Autodesk Inventor part; units mm, degrees
(part 4 of 6)
  line L818 (127.9253, -63.5518) -> (127.9253, -44.4306)
  spline S858 degree 2 poles (127.9253, -44.4306) (127.9253, -44.0268) (128.4872, -43.4824) (128.8735, -43.4824) knots 0 0 0 1 2 2 2
  spline S859 degree 2 poles (128.8735, -43.4824) (129.2773, -43.4824) (129.5583, -43.7458) knots 0 0 0 1 1 1
  spline S860 degree 2 poles (129.5583, -43.7458) (129.6636, -43.8512) (129.7163, -43.9741) knots 0 0 0 1 1 1
  line L819 (129.7163, -43.9741) -> (136.845, -59.2676)
  line L820 (136.845, -59.2676) -> (136.845, -44.4306)
  spline S861 degree 2 poles (136.845, -44.4306) (136.845, -44.0268) (137.3894, -43.4824) (137.7932, -43.4824) knots 0 0 0 1 2 2 2
  spline S862 degree 2 poles (137.7932, -43.4824) (138.197, -43.4824) (138.7414, -44.0268) (138.7414, -44.4306) knots 0 0 0 1 2 2 2
  line L821 (138.7414, -44.4306) -> (138.7414, -63.5694)
  spline S863 degree 2 poles (138.7414, -63.5694) (138.7414, -63.9381) (138.478, -64.2191) knots 0 0 0 1 1 1
  spline S864 degree 2 poles (138.478, -64.2191) (138.197, -64.5) (137.7932, -64.5) knots 0 0 0 1 1 1
  spline S865 degree 2 poles (137.7932, -64.5) (137.3894, -64.5) (137.126, -64.2191) knots 0 0 0 1 1 1
  spline S866 degree 2 poles (137.126, -64.2191) (136.9855, -64.0786) (136.8802, -63.8679) knots 0 0 0 1 1 1
  line L822 (136.8802, -63.8679) -> (129.8392, -48.6271)
  line L823 (129.8392, -48.6271) -> (129.8392, -63.5518)
  spline S867 degree 2 poles (165.7097, -44.4482) (165.7097, -44.0443) (166.2716, -43.5) (166.6579, -43.5) knots 0 0 0 1 2 2 2
  spline S868 degree 2 poles (166.6579, -43.5) (167.0617, -43.5) (167.6236, -44.0443) (167.6236, -44.4482) knots 0 0 0 1 2 2 2
  line L824 (167.6236, -44.4482) -> (167.6236, -63.5518)
  spline S869 degree 2 poles (167.6236, -63.5518) (167.6236, -63.9381) (167.0617, -64.5) (166.6579, -64.5) knots 0 0 0 1 2 2 2
  spline S870 degree 2 poles (166.6579, -64.5) (166.2716, -64.5) (165.7097, -63.9381) (165.7097, -63.5518) knots 0 0 0 1 2 2 2
  line L825 (165.7097, -63.5518) -> (165.7097, -44.4482)
  spline S871 degree 2 poles (-166.6579, -94.1789) (-166.2716, -94.1789) (-165.7097, -94.7408) (-165.7097, -95.1446) knots 0 0 0 1 2 2 2
  spline S872 degree 2 poles (-165.7097, -95.1446) (-165.7097, -95.5309) (-166.2716, -96.0928) (-166.6579, -96.0928) knots 0 0 0 1 2 2 2
  line L826 (-166.6579, -96.0928) -> (-169.836, -96.0928)
  line L827 (-169.836, -96.0928) -> (-170.8017, -99.7099)
  spline S873 degree 2 poles (-170.8017, -99.7099) (-170.8895, -100.0084) (-171.0826, -100.2191) knots 0 0 0 1 1 1
  spline S874 degree 2 poles (-171.0826, -100.2191) (-171.3636, -100.5) (-171.7499, -100.5) knots 0 0 0 1 1 1
  spline S875 degree 2 poles (-171.7499, -100.5) (-172.1537, -100.5) (-172.7156, -99.9381) (-172.7156, -99.5518) knots 0 0 0 1 2 2 2
  spline S876 degree 2 poles (-172.7156, -99.5518) (-172.7156, -99.4289) (-172.698, -99.3411) knots 0 0 0 1 1 1
  line L828 (-172.698, -99.3411) -> (-167.606, -80.3428)
  spline S877 degree 2 poles (-167.606, -80.3428) (-167.5358, -80.0268) (-167.3251, -79.7985) knots 0 0 0 1 1 1
  spline S878 degree 2 poles (-167.3251, -79.7985) (-167.0442, -79.5) (-166.6579, -79.5) knots 0 0 0 1 1 1
  spline S879 degree 2 poles (-166.6579, -79.5) (-166.2716, -79.5) (-165.9731, -79.7985) knots 0 0 0 1 1 1
  spline S880 degree 2 poles (-165.9731, -79.7985) (-165.7975, -80.0268) (-165.7273, -80.3428) knots 0 0 0 1 1 1
  line L829 (-165.7273, -80.3428) -> (-160.6353, -99.3411)
  spline S881 degree 2 poles (-160.6353, -99.3411) (-160.6178, -99.4289) (-160.6178, -99.5518) knots 0 0 0 1 1 1
  spline S882 degree 2 poles (-160.6178, -99.5518) (-160.6178, -99.9381) (-161.1796, -100.5) (-161.5659, -100.5) knots 0 0 0 1 2 2 2
  spline S883 degree 2 poles (-161.5659, -100.5) (-161.9698, -100.5) (-162.2331, -100.2191) knots 0 0 0 1 1 1
  spline S884 degree 2 poles (-162.2331, -100.2191) (-162.4438, -100.0084) (-162.5316, -99.7099) knots 0 0 0 1 1 1
  line L830 (-162.5316, -99.7099) -> (-166.6579, -84.2057)
  line L831 (-166.6579, -84.2057) -> (-169.3268, -94.1789)
  line L832 (-169.3268, -94.1789) -> (-166.6579, -94.1789)
  spline S885 degree 2 poles (-130.524, -97.7784) (-130.2606, -97.5151) (-129.8567, -97.5151) knots 0 0 0 1 1 1
  spline S886 degree 2 poles (-129.8567, -97.5151) (-129.4705, -97.5151) (-128.9086, -98.0594) (-128.9086, -98.4632) knots 0 0 0 1 2 2 2
  spline S887 degree 2 poles (-128.9086, -98.4632) (-128.9086, -98.8495) (-129.172, -99.1304) knots 0 0 0 1 1 1
  spline S888 degree 2 poles (-129.172, -99.1304) (-130.524, -100.5) (-132.3676, -100.5) knots 0 0 0 1 1 1
  spline S889 degree 2 poles (-132.3676, -100.5) (-134.2288, -100.5) (-136.8275, -97.8838) (-136.8275, -96.0401) knots 0 0 0 1 2 2 2
  line L833 (-136.8275, -96.0401) -> (-136.8275, -83.2751)
  spline S890 degree 2 poles (-136.8275, -83.2751) (-136.8275, -81.4314) (-134.2288, -78.8152) (-132.3676, -78.8152) knots 0 0 0 1 2 2 2
  spline S891 degree 2 poles (-132.3676, -78.8152) (-130.524, -78.8152) (-129.172, -80.1848) knots 0 0 0 1 1 1
  spline S892 degree 2 poles (-129.172, -80.1848) (-128.9086, -80.4833) (-128.9086, -80.852) knots 0 0 0 1 1 1
  spline S893 degree 2 poles (-128.9086, -80.852) (-128.9086, -81.2559) (-129.4705, -81.8177) (-129.8567, -81.8177) knots 0 0 0 1 2 2 2
  spline S894 degree 2 poles (-129.8567, -81.8177) (-130.2606, -81.8177) (-130.524, -81.5368) knots 0 0 0 1 1 1
  spline S895 degree 2 poles (-130.524, -81.5368) (-131.3317, -80.7467) (-132.3676, -80.7467) knots 0 0 0 1 1 1
  spline S896 degree 2 poles (-132.3676, -80.7467) (-133.4387, -80.7467) (-134.9136, -82.2391) (-134.9136, -83.2926) knots 0 0 0 1 2 2 2
  line L834 (-134.9136, -83.2926) -> (-134.9136, -96.0226)
  spline S897 degree 2 poles (-134.9136, -96.0226) (-134.9136, -97.0761) (-133.4387, -98.5686) (-132.3676, -98.5686) knots 0 0 0 1 2 2 2
  spline S898 degree 2 poles (-132.3676, -98.5686) (-131.3317, -98.5686) (-130.524, -97.7784) knots 0 0 0 1 1 1
  spline S899 degree 2 poles (-104.7759, -80.4482) (-104.7759, -80.0443) (-104.214, -79.5) (-103.8278, -79.5) knots 0 0 0 1 2 2 2
  spline S900 degree 2 poles (-103.8278, -79.5) (-103.4239, -79.5) (-102.862, -80.0443) (-102.862, -80.4482) knots 0 0 0 1 2 2 2
  line L835 (-102.862, -80.4482) -> (-102.862, -89.0343)
  line L836 (-102.862, -89.0343) -> (-97.1555, -89.0343)
  line L837 (-97.1555, -89.0343) -> (-97.1555, -80.4482)
  spline S901 degree 2 poles (-97.1555, -80.4482) (-97.1555, -80.0443) (-96.5936, -79.5) (-96.1898, -79.5) knots 0 0 0 1 2 2 2
  spline S902 degree 2 poles (-96.1898, -79.5) (-95.8035, -79.5) (-95.2416, -80.0443) (-95.2416, -80.4482) knots 0 0 0 1 2 2 2
  line L838 (-95.2416, -80.4482) -> (-95.2416, -99.5518)
  spline S903 degree 2 poles (-95.2416, -99.5518) (-95.2416, -99.9381) (-95.8035, -100.5) (-96.1898, -100.5) knots 0 0 0 1 2 2 2
  spline S904 degree 2 poles (-96.1898, -100.5) (-96.5936, -100.5) (-97.1555, -99.9381) (-97.1555, -99.5518) knots 0 0 0 1 2 2 2
  line L839 (-97.1555, -99.5518) -> (-97.1555, -90.9482)
  line L840 (-97.1555, -90.9482) -> (-102.862, -90.9482)
  line L841 (-102.862, -90.9482) -> (-102.862, -99.5518)
  spline S905 degree 2 poles (-102.862, -99.5518) (-102.862, -99.9381) (-103.4239, -100.5) (-103.8278, -100.5) knots 0 0 0 1 2 2 2
  spline S906 degree 2 poles (-103.8278, -100.5) (-104.214, -100.5) (-104.7759, -99.9381) (-104.7759, -99.5518) knots 0 0 0 1 2 2 2
  line L842 (-104.7759, -99.5518) -> (-104.7759, -80.4482)
  spline S907 degree 2 poles (-70.3364, -81.3963) (-70.7227, -81.3963) (-71.2846, -80.852) (-71.2846, -80.4482) knots 0 0 0 1 2 2 2
  spline S908 degree 2 poles (-71.2846, -80.4482) (-71.2846, -80.0443) (-70.7227, -79.5) (-70.3364, -79.5) knots 0 0 0 1 2 2 2
  line L843 (-70.3364, -79.5) -> (-63.3305, -79.5)
  spline S909 degree 2 poles (-63.3305, -79.5) (-62.9267, -79.5) (-62.3648, -80.0443) (-62.3648, -80.4482) knots 0 0 0 1 2 2 2
  spline S910 degree 2 poles (-62.3648, -80.4482) (-62.3648, -80.852) (-62.9267, -81.3963) (-63.3305, -81.3963) knots 0 0 0 1 2 2 2
  line L844 (-63.3305, -81.3963) -> (-65.8765, -81.3963)
  line L845 (-65.8765, -81.3963) -> (-65.8765, -99.5518)
  spline S911 degree 2 poles (-65.8765, -99.5518) (-65.8765, -99.9381) (-66.4208, -100.5) (-66.8247, -100.5) knots 0 0 0 1 2 2 2
  spline S912 degree 2 poles (-66.8247, -100.5) (-67.2285, -100.5) (-67.7904, -99.9381) (-67.7904, -99.5518) knots 0 0 0 1 2 2 2
  line L846 (-67.7904, -99.5518) -> (-67.7904, -81.3963)
  line L847 (-67.7904, -81.3963) -> (-70.3364, -81.3963)
  spline S913 degree 2 poles (-34.2903, -80.4482) (-34.2903, -80.0443) (-33.7284, -79.5) (-33.3421, -79.5) knots 0 0 0 1 2 2 2
  spline S914 degree 2 poles (-33.3421, -79.5) (-32.9383, -79.5) (-32.3764, -80.0443) (-32.3764, -80.4482) knots 0 0 0 1 2 2 2
  line L848 (-32.3764, -80.4482) -> (-32.3764, -99.5518)
  spline S915 degree 2 poles (-32.3764, -99.5518) (-32.3764, -99.9381) (-32.9383, -100.5) (-33.3421, -100.5) knots 0 0 0 1 2 2 2
  spline S916 degree 2 poles (-33.3421, -100.5) (-33.7284, -100.5) (-34.2903, -99.9381) (-34.2903, -99.5518) knots 0 0 0 1 2 2 2
  line L849 (-34.2903, -99.5518) -> (-34.2903, -80.4482)
  spline S917 degree 2 poles (-3.4941, -99.5518) (-3.4941, -99.9381) (-4.056, -100.5) (-4.4599, -100.5) knots 0 0 0 1 2 2 2
  spline S918 degree 2 poles (-4.4599, -100.5) (-4.8462, -100.5) (-5.408, -99.9381) (-5.408, -99.5518) knots 0 0 0 1 2 2 2
  line L850 (-5.408, -99.5518) -> (-5.408, -80.4306)
  spline S919 degree 2 poles (-5.408, -80.4306) (-5.408, -80.0268) (-4.8462, -79.4824) (-4.4599, -79.4824) knots 0 0 0 1 2 2 2
  spline S920 degree 2 poles (-4.4599, -79.4824) (-4.056, -79.4824) (-3.7751, -79.7458) knots 0 0 0 1 1 1
  spline S921 degree 2 poles (-3.7751, -79.7458) (-3.6697, -79.8512) (-3.6171, -79.9741) knots 0 0 0 1 1 1
  line L851 (-3.6171, -79.9741) -> (3.5117, -95.2676)
  line L852 (3.5117, -95.2676) -> (3.5117, -80.4306)
  spline S922 degree 2 poles (3.5117, -80.4306) (3.5117, -80.0268) (4.056, -79.4824) (4.4599, -79.4824) knots 0 0 0 1 2 2 2
  spline S923 degree 2 poles (4.4599, -79.4824) (4.8637, -79.4824) (5.408, -80.0268) (5.408, -80.4306) knots 0 0 0 1 2 2 2
  line L853 (5.408, -80.4306) -> (5.408, -99.5694)
  spline S924 degree 2 poles (5.408, -99.5694) (5.408, -99.9381) (5.1446, -100.2191) knots 0 0 0 1 1 1
  spline S925 degree 2 poles (5.1446, -100.2191) (4.8637, -100.5) (4.4599, -100.5) knots 0 0 0 1 1 1
  spline S926 degree 2 poles (4.4599, -100.5) (4.056, -100.5) (3.7926, -100.2191) knots 0 0 0 1 1 1
  spline S927 degree 2 poles (3.7926, -100.2191) (3.6522, -100.0786) (3.5468, -99.8679) knots 0 0 0 1 1 1
  line L854 (3.5468, -99.8679) -> (-3.4941, -84.6271)
  line L855 (-3.4941, -84.6271) -> (-3.4941, -99.5518)
  spline S928 degree 2 poles (28.8822, -80.1497) (28.8822, -79.7458) (29.4441, -79.1839) (29.8304, -79.1839) knots 0 0 0 1 2 2 2
  spline S929 degree 2 poles (29.8304, -79.1839) (30.2343, -79.1839) (30.7961, -79.7458) (30.7961, -80.1497) knots 0 0 0 1 2 2 2
  line L856 (30.7961, -80.1497) -> (30.7961, -96.0401)
  spline S930 degree 2 poles (30.7961, -96.0401) (30.7961, -97.0936) (32.2886, -98.5861) (33.3421, -98.5861) knots 0 0 0 1 2 2 2
  spline S931 degree 2 poles (33.3421, -98.5861) (34.3956, -98.5861) (35.8881, -97.0936) (35.8881, -96.0401) knots 0 0 0 1 2 2 2
  line L857 (35.8881, -96.0401) -> (35.8881, -80.1497)
  spline S932 degree 2 poles (35.8881, -80.1497) (35.8881, -79.7458) (36.4324, -79.1839) (36.8363, -79.1839) knots 0 0 0 1 2 2 2
  spline S933 degree 2 poles (36.8363, -79.1839) (37.2401, -79.1839) (37.802, -79.7458) (37.802, -80.1497) knots 0 0 0 1 2 2 2
  line L858 (37.802, -80.1497) -> (37.802, -96.0401)
  spline S934 degree 2 poles (37.802, -96.0401) (37.802, -97.8838) (35.1858, -100.5) (33.3421, -100.5) knots 0 0 0 1 2 2 2
  spline S935 degree 2 poles (33.3421, -100.5) (31.4985, -100.5) (28.8822, -97.8838) (28.8822, -96.0401) knots 0 0 0 1 2 2 2
  line L859 (28.8822, -96.0401) -> (28.8822, -80.1497)
  spline S936 degree 2 poles (31.0244, -74.0744) (31.5511, -74.0744) (32.3062, -74.8294) (32.3062, -75.3562) knots 0 0 0 1 2 2 2
  spline S937 degree 2 poles (32.3062, -75.3562) (32.3062, -75.8829) (31.5511, -76.6204) (31.0244, -76.6204) knots 0 0 0 1 2 2 2
  spline S938 degree 2 poles (31.0244, -76.6204) (30.4976, -76.6204) (29.7602, -75.8829) (29.7602, -75.3562) knots 0 0 0 1 2 2 2
  spline S939 degree 2 poles (29.7602, -75.3562) (29.7602, -74.8294) (30.4976, -74.0744) (31.0244, -74.0744) knots 0 0 0 1 2 2 2
  spline S940 degree 2 poles (35.6598, -74.0744) (36.1866, -74.0744) (36.9416, -74.8294) (36.9416, -75.3562) knots 0 0 0 1 2 2 2
  spline S941 degree 2 poles (36.9416, -75.3562) (36.9416, -75.8829) (36.1866, -76.6204) (35.6598, -76.6204) knots 0 0 0 1 2 2 2
  spline S942 degree 2 poles (35.6598, -76.6204) (35.1331, -76.6204) (34.3956, -75.8829) (34.3956, -75.3562) knots 0 0 0 1 2 2 2
  spline S943 degree 2 poles (34.3956, -75.3562) (34.3956, -74.8294) (35.1331, -74.0744) (35.6598, -74.0744) knots 0 0 0 1 2 2 2
  spline S944 degree 2 poles (63.1725, -99.5518) (63.1725, -99.9381) (62.6106, -100.5) (62.2068, -100.5) knots 0 0 0 1 2 2 2
  spline S945 degree 2 poles (62.2068, -100.5) (61.8205, -100.5) (61.2586, -99.9381) (61.2586, -99.5518) knots 0 0 0 1 2 2 2
  line L860 (61.2586, -99.5518) -> (61.2586, -80.4306)
  spline S946 degree 2 poles (61.2586, -80.4306) (61.2586, -80.0268) (61.8205, -79.4824) (62.2068, -79.4824) knots 0 0 0 1 2 2 2
  spline S947 degree 2 poles (62.2068, -79.4824) (62.6106, -79.4824) (62.8916, -79.7458) knots 0 0 0 1 1 1
  spline S948 degree 2 poles (62.8916, -79.7458) (62.9969, -79.8512) (63.0496, -79.9741) knots 0 0 0 1 1 1
  line L861 (63.0496, -79.9741) -> (70.1784, -95.2676)
  line L862 (70.1784, -95.2676) -> (70.1784, -80.4306)
  spline S949 degree 2 poles (70.1784, -80.4306) (70.1784, -80.0268) (70.7227, -79.4824) (71.1265, -79.4824) knots 0 0 0 1 2 2 2
  spline S950 degree 2 poles (71.1265, -79.4824) (71.5304, -79.4824) (72.0747, -80.0268) (72.0747, -80.4306) knots 0 0 0 1 2 2 2
  line L863 (72.0747, -80.4306) -> (72.0747, -99.5694)
  spline S951 degree 2 poles (72.0747, -99.5694) (72.0747, -99.9381) (71.8113, -100.2191) knots 0 0 0 1 1 1
  spline S952 degree 2 poles (71.8113, -100.2191) (71.5304, -100.5) (71.1265, -100.5) knots 0 0 0 1 1 1
  spline S953 degree 2 poles (71.1265, -100.5) (70.7227, -100.5) (70.4593, -100.2191) knots 0 0 0 1 1 1
  spline S954 degree 2 poles (70.4593, -100.2191) (70.3188, -100.0786) (70.2135, -99.8679) knots 0 0 0 1 1 1
  line L864 (70.2135, -99.8679) -> (63.1725, -84.6271)
  line L865 (63.1725, -84.6271) -> (63.1725, -99.5518)
  spline S955 degree 2 poles (99.0431, -80.4482) (99.0431, -80.0443) (99.6049, -79.5) (99.9912, -79.5) knots 0 0 0 1 2 2 2
  spline S956 degree 2 poles (99.9912, -79.5) (100.3951, -79.5) (100.9569, -80.0443) (100.9569, -80.4482) knots 0 0 0 1 2 2 2
  line L866 (100.9569, -80.4482) -> (100.9569, -99.5518)
  spline S957 degree 2 poles (100.9569, -99.5518) (100.9569, -99.9381) (100.3951, -100.5) (99.9912, -100.5) knots 0 0 0 1 2 2 2
  spline S958 degree 2 poles (99.9912, -100.5) (99.6049, -100.5) (99.0431, -99.9381) (99.0431, -99.5518) knots 0 0 0 1 2 2 2
  line L867 (99.0431, -99.5518) -> (99.0431, -80.4482)
  spline S959 degree 2 poles (130.1552, -80.4482) (130.1552, -80.0443) (130.7171, -79.5) (131.1034, -79.5) knots 0 0 0 1 2 2 2
  line L868 (131.1034, -79.5) -> (137.1787, -79.5)
  spline S960 degree 2 poles (137.1787, -79.5) (137.5649, -79.5) (138.1268, -80.0443) (138.1268, -80.4482) knots 0 0 0 1 2 2 2
  spline S961 degree 2 poles (138.1268, -80.4482) (138.1268, -80.8344) (137.5649, -81.3963) (137.1787, -81.3963) knots 0 0 0 1 2 2 2
  line L869 (137.1787, -81.3963) -> (132.0691, -81.3963)
  line L870 (132.0691, -81.3963) -> (132.0691, -89.0343)
  line L871 (132.0691, -89.0343) -> (136.1954, -89.0343)
  spline S962 degree 2 poles (136.1954, -89.0343) (136.5992, -89.0343) (137.1611, -89.5962) (137.1611, -90) knots 0 0 0 1 2 2 2
  spline S963 degree 2 poles (137.1611, -90) (137.1611, -90.3863) (136.5992, -90.9482) (136.1954, -90.9482) knots 0 0 0 1 2 2 2
  line L872 (136.1954, -90.9482) -> (132.0691, -90.9482)
  line L873 (132.0691, -90.9482) -> (132.0691, -98.5861)
  line L874 (132.0691, -98.5861) -> (137.1787, -98.5861)
  spline S964 degree 2 poles (137.1787, -98.5861) (137.5649, -98.5861) (138.1268, -99.148) (138.1268, -99.5518) knots 0 0 0 1 2 2 2
  spline S965 degree 2 poles (138.1268, -99.5518) (138.1268, -99.9206) (137.5649, -100.5) (137.1787, -100.5) knots 0 0 0 1 2 2 2
  line L875 (137.1787, -100.5) -> (131.1034, -100.5)
  spline S966 degree 2 poles (131.1034, -100.5) (130.7171, -100.5) (130.1552, -99.9381) (130.1552, -99.5518) knots 0 0 0 1 2 2 2
  line L876 (130.1552, -99.5518) -> (130.1552, -80.4482)
  spline S967 degree 2 poles (164.1207, -80.4482) (164.1207, -80.0443) (164.6826, -79.5) (165.0688, -79.5) knots 0 0 0 1 2 2 2
  spline S968 degree 2 poles (165.0688, -79.5) (165.4727, -79.5) (166.0346, -80.0443) (166.0346, -80.4482) knots 0 0 0 1 2 2 2
  line L877 (166.0346, -80.4482) -> (166.0346, -98.5861)
  line L878 (166.0346, -98.5861) -> (170.4944, -98.5861)
  spline S969 degree 2 poles (170.4944, -98.5861) (170.8807, -98.5861) (171.4426, -99.148) (171.4426, -99.5518) knots 0 0 0 1 2 2 2
  spline S970 degree 2 poles (171.4426, -99.5518) (171.4426, -99.9381) (170.8807, -100.5) (170.4944, -100.5) knots 0 0 0 1 2 2 2
  line L879 (170.4944, -100.5) -> (165.0688, -100.5)
  spline S971 degree 2 poles (165.0688, -100.5) (164.6826, -100.5) (164.1207, -99.9381) (164.1207, -99.5518) knots 0 0 0 1 2 2 2
  line L880 (164.1207, -99.5518) -> (164.1207, -80.4482)
  spline S972 degree 2 poles (-170.4417, -117.3963) (-170.8456, -117.3963) (-171.4075, -116.852) (-171.4075, -116.4482) knots 0 0 0 1 2 2 2
  spline S973 degree 2 poles (-171.4075, -116.4482) (-171.4075, -116.0443) (-170.8456, -115.5) (-170.4417, -115.5) knots 0 0 0 1 2 2 2
  line L881 (-170.4417, -115.5) -> (-163.1198, -115.5)
  spline S974 degree 2 poles (-163.1198, -115.5) (-162.7336, -115.5) (-162.1717, -116.0443) (-162.1717, -116.4482) knots 0 0 0 1 2 2 2
  spline S975 degree 2 poles (-162.1717, -116.4482) (-162.1717, -116.6413) (-162.2419, -116.8169) knots 0 0 0 1 1 1
  line L882 (-162.2419, -116.8169) -> (-169.0546, -134.5861)
  line L883 (-169.0546, -134.5861) -> (-163.1198, -134.5861)
  spline S976 degree 2 poles (-163.1198, -134.5861) (-162.7336, -134.5861) (-162.1717, -135.148) (-162.1717, -135.5518) knots 0 0 0 1 2 2 2
  spline S977 degree 2 poles (-162.1717, -135.5518) (-162.1717, -135.9206) (-162.7336, -136.5) (-163.1198, -136.5) knots 0 0 0 1 2 2 2
  line L884 (-163.1198, -136.5) -> (-170.4417, -136.5)
  spline S978 degree 2 poles (-170.4417, -136.5) (-170.828, -136.5) (-171.3899, -135.9206) (-171.3899, -135.5518) knots 0 0 0 1 2 2 2
  spline S979 degree 2 poles (-171.3899, -135.5518) (-171.3899, -135.306) (-171.3021, -135.1129) knots 0 0 0 1 1 1
  line L885 (-171.3021, -135.1129) -> (-164.5245, -117.3963)
  line L886 (-164.5245, -117.3963) -> (-170.4417, -117.3963)
  spline S980 degree 2 poles (-133.3246, -130.1789) (-132.9383, -130.1789) (-132.3764, -130.7408) (-132.3764, -131.1446) knots 0 0 0 1 2 2 2
  spline S981 degree 2 poles (-132.3764, -131.1446) (-132.3764, -131.5309) (-132.9383, -132.0928) (-133.3246, -132.0928) knots 0 0 0 1 2 2 2
  line L887 (-133.3246, -132.0928) -> (-136.5026, -132.0928)
  line L888 (-136.5026, -132.0928) -> (-137.4684, -135.7099)
  spline S982 degree 2 poles (-137.4684, -135.7099) (-137.5562, -136.0084) (-137.7493, -136.2191) knots 0 0 0 1 1 1
  spline S983 degree 2 poles (-137.7493, -136.2191) (-138.0302, -136.5) (-138.4165, -136.5) knots 0 0 0 1 1 1
  spline S984 degree 2 poles (-138.4165, -136.5) (-138.8204, -136.5) (-139.3822, -135.9381) (-139.3822, -135.5518) knots 0 0 0 1 2 2 2
  spline S985 degree 2 poles (-139.3822, -135.5518) (-139.3822, -135.4289) (-139.3647, -135.3411) knots 0 0 0 1 1 1
  line L889 (-139.3647, -135.3411) -> (-134.2727, -116.3428)
  spline S986 degree 2 poles (-134.2727, -116.3428) (-134.2025, -116.0268) (-133.9918, -115.7985) knots 0 0 0 1 1 1
  spline S987 degree 2 poles (-133.9918, -115.7985) (-133.7108, -115.5) (-133.3246, -115.5) knots 0 0 0 1 1 1
  spline S988 degree 2 poles (-133.3246, -115.5) (-132.9383, -115.5) (-132.6398, -115.7985) knots 0 0 0 1 1 1
  spline S989 degree 2 poles (-132.6398, -115.7985) (-132.4642, -116.0268) (-132.394, -116.3428) knots 0 0 0 1 1 1
  line L890 (-132.394, -116.3428) -> (-127.302, -135.3411)
  spline S990 degree 2 poles (-127.302, -135.3411) (-127.2844, -135.4289) (-127.2844, -135.5518) knots 0 0 0 1 1 1
  spline S991 degree 2 poles (-127.2844, -135.5518) (-127.2844, -135.9381) (-127.8463, -136.5) (-128.2326, -136.5) knots 0 0 0 1 2 2 2
  spline S992 degree 2 poles (-128.2326, -136.5) (-128.6364, -136.5) (-128.8998, -136.2191) knots 0 0 0 1 1 1
  spline S993 degree 2 poles (-128.8998, -136.2191) (-129.1105, -136.0084) (-129.1983, -135.7099) knots 0 0 0 1 1 1
  line L891 (-129.1983, -135.7099) -> (-133.3246, -120.2057)
  line L892 (-133.3246, -120.2057) -> (-135.9935, -130.1789)
  line L893 (-135.9935, -130.1789) -> (-133.3246, -130.1789)
  spline S994 degree 2 poles (-131.0068, -110.3905) (-130.4801, -110.3905) (-129.7426, -111.1455) (-129.7426, -111.6722) knots 0 0 0 1 2 2 2
  spline S995 degree 2 poles (-129.7426, -111.6722) (-129.7426, -112.199) (-130.4801, -112.9365) (-131.0068, -112.9365) knots 0 0 0 1 2 2 2
  spline S996 degree 2 poles (-131.0068, -112.9365) (-131.5336, -112.9365) (-132.2886, -112.199) (-132.2886, -111.6722) knots 0 0 0 1 2 2 2
  spline S997 degree 2 poles (-132.2886, -111.6722) (-132.2886, -111.1455) (-131.5336, -110.3905) (-131.0068, -110.3905) knots 0 0 0 1 2 2 2
  spline S998 degree 2 poles (-135.6423, -110.3905) (-135.1155, -110.3905) (-134.3605, -111.1455) (-134.3605, -111.6722) knots 0 0 0 1 2 2 2
  spline S999 degree 2 poles (-134.3605, -111.6722) (-134.3605, -112.199) (-135.1155, -112.9365) (-135.6423, -112.9365) knots 0 0 0 1 2 2 2
  spline S1000 degree 2 poles (-135.6423, -112.9365) (-136.169, -112.9365) (-136.9065, -112.199) (-136.9065, -111.6722) knots 0 0 0 1 2 2 2
  spline S1001 degree 2 poles (-136.9065, -111.6722) (-136.9065, -111.1455) (-136.169, -110.3905) (-135.6423, -110.3905) knots 0 0 0 1 2 2 2
  spline S1002 degree 2 poles (-103.4941, -135.5518) (-103.4941, -135.9381) (-104.056, -136.5) (-104.4599, -136.5) knots 0 0 0 1 2 2 2
  spline S1003 degree 2 poles (-104.4599, -136.5) (-104.8462, -136.5) (-105.408, -135.9381) (-105.408, -135.5518) knots 0 0 0 1 2 2 2
  line L894 (-105.408, -135.5518) -> (-105.408, -116.4306)
  spline S1004 degree 2 poles (-105.408, -116.4306) (-105.408, -116.0268) (-104.8462, -115.4824) (-104.4599, -115.4824) knots 0 0 0 1 2 2 2
  spline S1005 degree 2 poles (-104.4599, -115.4824) (-104.056, -115.4824) (-103.7751, -115.7458) knots 0 0 0 1 1 1
  spline S1006 degree 2 poles (-103.7751, -115.7458) (-103.6697, -115.8512) (-103.6171, -115.9741) knots 0 0 0 1 1 1
  line L895 (-103.6171, -115.9741) -> (-96.4883, -131.2676)
  line L896 (-96.4883, -131.2676) -> (-96.4883, -116.4306)
  spline S1007 degree 2 poles (-96.4883, -116.4306) (-96.4883, -116.0268) (-95.944, -115.4824) (-95.5401, -115.4824) knots 0 0 0 1 2 2 2
  spline S1008 degree 2 poles (-95.5401, -115.4824) (-95.1363, -115.4824) (-94.592, -116.0268) (-94.592, -116.4306) knots 0 0 0 1 2 2 2
  line L897 (-94.592, -116.4306) -> (-94.592, -135.5694)
  spline S1009 degree 2 poles (-94.592, -135.5694) (-94.592, -135.9381) (-94.8554, -136.2191) knots 0 0 0 1 1 1
  spline S1010 degree 2 poles (-94.8554, -136.2191) (-95.1363, -136.5) (-95.5401, -136.5) knots 0 0 0 1 1 1
  spline S1011 degree 2 poles (-95.5401, -136.5) (-95.944, -136.5) (-96.2074, -136.2191) knots 0 0 0 1 1 1
  spline S1012 degree 2 poles (-96.2074, -136.2191) (-96.3478, -136.0786) (-96.4532, -135.8679) knots 0 0 0 1 1 1
  line L898 (-96.4532, -135.8679) -> (-103.4941, -120.6271)
  line L899 (-103.4941, -120.6271) -> (-103.4941, -135.5518)
  spline S1013 degree 2 poles (-67.6236, -116.4482) (-67.6236, -116.0443) (-67.0617, -115.5) (-66.6754, -115.5) knots 0 0 0 1 2 2 2
  spline S1014 degree 2 poles (-66.6754, -115.5) (-66.2716, -115.5) (-65.7097, -116.0443) (-65.7097, -116.4482) knots 0 0 0 1 2 2 2
  line L900 (-65.7097, -116.4482) -> (-65.7097, -135.5518)
  spline S1015 degree 2 poles (-65.7097, -135.5518) (-65.7097, -135.9381) (-66.2716, -136.5) (-66.6754, -136.5) knots 0 0 0 1 2 2 2
  spline S1016 degree 2 poles (-66.6754, -136.5) (-67.0617, -136.5) (-67.6236, -135.9381) (-67.6236, -135.5518) knots 0 0 0 1 2 2 2
  line L901 (-67.6236, -135.5518) -> (-67.6236, -116.4482)
  spline S1017 degree 2 poles (-36.5114, -116.4482) (-36.5114, -116.0443) (-35.9496, -115.5) (-35.5633, -115.5) knots 0 0 0 1 2 2 2
  line L902 (-35.5633, -115.5) -> (-29.488, -115.5)
  spline S1018 degree 2 poles (-29.488, -115.5) (-29.1017, -115.5) (-28.5399, -116.0443) (-28.5399, -116.4482) knots 0 0 0 1 2 2 2
  spline S1019 degree 2 poles (-28.5399, -116.4482) (-28.5399, -116.8344) (-29.1017, -117.3963) (-29.488, -117.3963) knots 0 0 0 1 2 2 2
  line L903 (-29.488, -117.3963) -> (-34.5975, -117.3963)
  line L904 (-34.5975, -117.3963) -> (-34.5975, -125.0343)
  line L905 (-34.5975, -125.0343) -> (-30.4713, -125.0343)
  spline S1020 degree 2 poles (-30.4713, -125.0343) (-30.0674, -125.0343) (-29.5056, -125.5962) (-29.5056, -126) knots 0 0 0 1 2 2 2
  spline S1021 degree 2 poles (-29.5056, -126) (-29.5056, -126.3863) (-30.0674, -126.9482) (-30.4713, -126.9482) knots 0 0 0 1 2 2 2
  line L906 (-30.4713, -126.9482) -> (-34.5975, -126.9482)
  line L907 (-34.5975, -126.9482) -> (-34.5975, -134.5861)
  line L908 (-34.5975, -134.5861) -> (-29.488, -134.5861)
  spline S1022 degree 2 poles (-29.488, -134.5861) (-29.1017, -134.5861) (-28.5399, -135.148) (-28.5399, -135.5518) knots 0 0 0 1 2 2 2
  spline S1023 degree 2 poles (-28.5399, -135.5518) (-28.5399, -135.9206) (-29.1017, -136.5) (-29.488, -136.5) knots 0 0 0 1 2 2 2
  line L909 (-29.488, -136.5) -> (-35.5633, -136.5)
  spline S1024 degree 2 poles (-35.5633, -136.5) (-35.9496, -136.5) (-36.5114, -135.9381) (-36.5114, -135.5518) knots 0 0 0 1 2 2 2
  line L910 (-36.5114, -135.5518) -> (-36.5114, -116.4482)
  spline S1025 degree 2 poles (1.4837, -127.8436) (1.9227, -127.7207) (2.3089, -127.352) knots 0 0 0 1 1 1
  spline S1026 degree 2 poles (2.3089, -127.352) (2.8708, -126.7901) (2.8708, -126) knots 0 0 0 1 1 1
  line L911 (2.8708, -126) -> (2.8708, -119.3102)
  spline S1027 degree 2 poles (2.8708, -119.3102) (2.8708, -118.5201) (1.7471, -117.3963) (0.9569, -117.3963) knots 0 0 0 1 2 2 2
  line L912 (0.9569, -117.3963) -> (-2.2212, -117.3963)
  line L913 (-2.2212, -117.3963) -> (-2.2212, -135.5518)
  spline S1028 degree 2 poles (-2.2212, -135.5518) (-2.2212, -135.9381) (-2.783, -136.5) (-3.1869, -136.5) knots 0 0 0 1 2 2 2
  spline S1029 degree 2 poles (-3.1869, -136.5) (-3.5732, -136.5) (-4.135, -135.9381) (-4.135, -135.5518) knots 0 0 0 1 2 2 2
  line L914 (-4.135, -135.5518) -> (-4.135, -116.4482)
  spline S1030 degree 2 poles (-4.135, -116.4482) (-4.135, -116.0443) (-3.5732, -115.5) (-3.1869, -115.5) knots 0 0 0 1 2 2 2
  line L915 (-3.1869, -115.5) -> (0.9569, -115.5)
  spline S1031 degree 2 poles (0.9569, -115.5) (2.5372, -115.5) (4.7847, -117.7299) (4.7847, -119.3102) knots 0 0 0 1 2 2 2
  line L916 (4.7847, -119.3102) -> (4.7847, -126)
  spline S1032 degree 2 poles (4.7847, -126) (4.7847, -127.5627) (3.661, -128.6865) knots 0 0 0 1 1 1
  spline S1033 degree 2 poles (3.661, -128.6865) (3.3098, -129.0376) (2.9235, -129.2659) knots 0 0 0 1 1 1
  line L917 (2.9235, -129.2659) -> (5.3115, -135.1304)
  spline S1034 degree 2 poles (5.3115, -135.1304) (5.4168, -135.3411) (5.4168, -135.5518) knots 0 0 0 1 1 1
  spline S1035 degree 2 poles (5.4168, -135.5518) (5.4168, -135.6923) (5.3641, -135.8328) knots 0 0 0 1 1 1
  spline S1036 degree 2 poles (5.3641, -135.8328) (5.2412, -136.2191) (4.8901, -136.3946) knots 0 0 0 1 1 1
  spline S1037 degree 2 poles (4.8901, -136.3946) (4.6793, -136.5) (4.4686, -136.5) knots 0 0 0 1 1 1
  spline S1038 degree 2 poles (4.4686, -136.5) (4.3106, -136.5) (4.1702, -136.4649) knots 0 0 0 1 1 1
  spline S1039 degree 2 poles (4.1702, -136.4649) (3.7839, -136.342) (3.6083, -135.9732) knots 0 0 0 1 1 1
  line L918 (3.6083, -135.9732) -> (0.8867, -129.2308)
  spline S1040 degree 2 poles (0.8867, -129.2308) (0.7638, -129.0201) (0.7638, -128.7567) knots 0 0 0 1 1 1
  spline S1041 degree 2 poles (0.7638, -128.7567) (0.7638, -128.3704) (1.0623, -128.0719) knots 0 0 0 1 1 1
  spline S1042 degree 2 poles (1.0623, -128.0719) (1.2379, -127.8963) (1.4837, -127.8436) knots 0 0 0 1 1 1
  spline S1043 degree 2 poles (38.118, -132.0577) (38.118, -133.9013) (36.8011, -135.2007) knots 0 0 0 1 1 1
  spline S1044 degree 2 poles (36.8011, -135.2007) (35.6423, -136.3946) (34.0445, -136.5) knots 0 0 0 1 1 1
  spline S1045 degree 2 poles (34.0445, -136.5) (33.5704, -136.5) (33.0261, -135.9381) (33.0261, -135.5518) knots 0 0 0 1 2 2 2
  spline S1046 degree 2 poles (33.0261, -135.5518) (33.0261, -135.148) (33.307, -134.8671) knots 0 0 0 1 1 1
  spline S1047 degree 2 poles (33.307, -134.8671) (33.5353, -134.6212) (33.8864, -134.5861) knots 0 0 0 1 1 1
  spline S1048 degree 2 poles (33.8864, -134.5861) (34.7995, -134.5159) (35.4491, -133.8487) knots 0 0 0 1 1 1
  spline S1049 degree 2 poles (35.4491, -133.8487) (36.2042, -133.1112) (36.2042, -132.0577) knots 0 0 0 1 1 1
  line L919 (36.2042, -132.0577) -> (36.2042, -129.4415)
  spline S1050 degree 2 poles (36.2042, -129.4415) (36.2042, -128.4055) (35.4491, -127.6505) knots 0 0 0 1 1 1
  spline S1051 degree 2 poles (35.4491, -127.6505) (34.8521, -127.036) (34.0445, -126.9306) knots 0 0 0 1 1 1
  spline S1052 degree 2 poles (34.0445, -126.9306) (33.5704, -126.9306) (33.307, -126.6497) knots 0 0 0 1 1 1
  spline S1053 degree 2 poles (33.307, -126.6497) (33.0261, -126.3687) (33.0261, -125.9824) knots 0 0 0 1 1 1
  line L920 (33.0261, -125.9824) -> (33.0261, -125.9649)
  spline S1054 degree 2 poles (33.0261, -125.9649) (33.0261, -125.561) (33.307, -125.2801) knots 0 0 0 1 1 1
  spline S1055 degree 2 poles (33.307, -125.2801) (33.5704, -124.9992) (34.0445, -124.9992) knots 0 0 0 1 1 1
  spline S1056 degree 2 poles (34.0445, -124.9992) (34.8521, -124.8938) (35.4491, -124.2968) knots 0 0 0 1 1 1
  spline S1057 degree 2 poles (35.4491, -124.2968) (36.2042, -123.5418) (36.2042, -122.4883) knots 0 0 0 1 1 1
  line L921 (36.2042, -122.4883) -> (36.2042, -119.9072)
  spline S1058 degree 2 poles (36.2042, -119.9072) (36.2042, -118.8712) (35.4491, -118.1162) knots 0 0 0 1 1 1
  spline S1059 degree 2 poles (35.4491, -118.1162) (34.7995, -117.4666) (33.8864, -117.3788) knots 0 0 0 1 1 1
  spline S1060 degree 2 poles (33.8864, -117.3788) (33.5353, -117.3436) (33.307, -117.0978) knots 0 0 0 1 1 1
  spline S1061 degree 2 poles (33.307, -117.0978) (33.0261, -116.8344) (33.0261, -116.4306) knots 0 0 0 1 1 1
  spline S1062 degree 2 poles (33.0261, -116.4306) (33.0261, -116.0268) (33.5704, -115.4824) (34.0445, -115.4824) knots 0 0 0 1 2 2 2
  spline S1063 degree 2 poles (34.0445, -115.4824) (35.6423, -115.5878) (36.8011, -116.7642) knots 0 0 0 1 1 1
  spline S1064 degree 2 poles (36.8011, -116.7642) (38.118, -118.0635) (38.118, -119.9072) knots 0 0 0 1 1 1
  line L922 (38.118, -119.9072) -> (38.118, -122.4883)
  spline S1065 degree 2 poles (38.118, -122.4883) (38.118, -124.6656) (36.45, -125.9824) knots 0 0 0 1 1 1
  spline S1066 degree 2 poles (36.45, -125.9824) (38.118, -127.2818) (38.118, -129.4415) knots 0 0 0 1 1 1
  line L923 (38.118, -129.4415) -> (38.118, -132.0577)
  spline S1067 degree 2 poles (29.1983, -116.4306) (29.1983, -116.0268) (29.7602, -115.4824) (30.1465, -115.4824) knots 0 0 0 1 2 2 2
  spline S1068 degree 2 poles (30.1465, -115.4824) (30.5503, -115.4824) (31.1122, -116.0268) (31.1122, -116.4306) knots 0 0 0 1 2 2 2
  line L924 (31.1122, -116.4306) -> (31.1122, -135.5343)
  spline S1069 degree 2 poles (31.1122, -135.5343) (31.1122, -135.9206) (30.5503, -136.4824) (30.1465, -136.4824) knots 0 0 0 1 2 2 2
  spline S1070 degree 2 poles (30.1465, -136.4824) (29.7602, -136.4824) (29.1983, -135.9206) (29.1983, -135.5343) knots 0 0 0 1 2 2 2
  line L925 (29.1983, -135.5343) -> (29.1983, -116.4306)
  spline S1071 degree 2 poles (64.1997, -115.6405) (64.4455, -115.4824) (64.7616, -115.4824) knots 0 0 0 1 1 1
  spline S1072 degree 2 poles (64.7616, -115.4824) (65.1479, -115.4824) (65.7097, -116.0443) (65.7097, -116.4306) knots 0 0 0 1 2 2 2
  spline S1073 degree 2 poles (65.7097, -116.4306) (65.7097, -116.8344) (65.4463, -117.0978) knots 0 0 0 1 1 1
  spline S1074 degree 2 poles (65.4463, -117.0978) (65.3586, -117.1681) (65.2883, -117.2383) knots 0 0 0 1 1 1
  spline S1075 degree 2 poles (65.2883, -117.2383) (65.0601, -117.3788) (64.8669, -117.5719) knots 0 0 0 1 1 1
  spline S1076 degree 2 poles (64.8669, -117.5719) (64.1295, -118.3269) (64.1295, -119.3804) knots 0 0 0 1 1 1
  line L926 (64.1295, -119.3804) -> (64.1295, -132.602)
  spline S1077 degree 2 poles (64.1295, -132.602) (64.1295, -133.6555) (64.8669, -134.393) knots 0 0 0 1 1 1
  spline S1078 degree 2 poles (64.8669, -134.393) (65.0601, -134.5861) (65.2883, -134.7266) knots 0 0 0 1 1 1
  spline S1079 degree 2 poles (65.2883, -134.7266) (65.3586, -134.7793) (65.4288, -134.8495) knots 0 0 0 1 1 1
  spline S1080 degree 2 poles (65.4288, -134.8495) (65.7097, -135.1304) (65.7097, -135.5343) knots 0 0 0 1 1 1
  spline S1081 degree 2 poles (65.7097, -135.5343) (65.7097, -135.9206) (65.1479, -136.4824) (64.7616, -136.4824) knots 0 0 0 1 2 2 2
  spline S1082 degree 2 poles (64.7616, -136.4824) (64.4631, -136.4824) (64.2348, -136.342) knots 0 0 0 1 1 1
  spline S1083 degree 2 poles (64.2348, -136.342) (63.8485, -136.0786) (63.5149, -135.745) knots 0 0 0 1 1 1
  spline S1084 degree 2 poles (63.5149, -135.745) (62.2156, -134.4457) (62.2156, -132.602) knots 0 0 0 1 1 1
  line L927 (62.2156, -132.602) -> (62.2156, -119.3804)
  spline S1085 degree 2 poles (62.2156, -119.3804) (62.2156, -117.5192) (63.5149, -116.2199) knots 0 0 0 1 1 1
  spline S1086 degree 2 poles (63.5149, -116.2199) (63.8485, -115.8863) (64.1997, -115.6405) knots 0 0 0 1 1 1
  spline S1087 degree 2 poles (68.1679, -117.3085) (68.0275, -117.2383) (67.9045, -117.1154) knots 0 0 0 1 1 1
  spline S1088 degree 2 poles (67.9045, -117.1154) (67.6236, -116.8344) (67.6236, -116.4482) knots 0 0 0 1 1 1
  spline S1089 degree 2 poles (67.6236, -116.4482) (67.6236, -116.0443) (68.1855, -115.4824) (68.5718, -115.4824) knots 0 0 0 1 2 2 2
  spline S1090 degree 2 poles (68.5718, -115.4824) (68.8878, -115.4824) (69.1512, -115.658) knots 0 0 0 1 1 1
  spline S1091 degree 2 poles (69.1512, -115.658) (69.5024, -115.9038) (69.8184, -116.2199) knots 0 0 0 1 1 1
  spline S1092 degree 2 poles (69.8184, -116.2199) (71.1178, -117.5192) (71.1178, -119.3804) knots 0 0 0 1 1 1
  line L928 (71.1178, -119.3804) -> (71.1178, -132.602)
  spline S1093 degree 2 poles (71.1178, -132.602) (71.1178, -134.4457) (69.8184, -135.745) knots 0 0 0 1 1 1
  spline S1094 degree 2 poles (69.8184, -135.745) (69.4673, -136.0962) (69.081, -136.3595) knots 0 0 0 1 1 1
  spline S1095 degree 2 poles (69.081, -136.3595) (68.8703, -136.5) (68.5718, -136.5) knots 0 0 0 1 1 1
  spline S1096 degree 2 poles (68.5718, -136.5) (68.1855, -136.5) (67.6236, -135.9206) (67.6236, -135.5518) knots 0 0 0 1 2 2 2
  spline S1097 degree 2 poles (67.6236, -135.5518) (67.6236, -135.148) (67.9045, -134.8671) knots 0 0 0 1 1 1
  spline S1098 degree 2 poles (67.9045, -134.8671) (67.9748, -134.7968) (68.045, -134.7441) knots 0 0 0 1 1 1
  spline S1099 degree 2 poles (68.045, -134.7441) (68.2557, -134.6037) (68.4664, -134.393) knots 0 0 0 1 1 1
  spline S1100 degree 2 poles (68.4664, -134.393) (69.2214, -133.6555) (69.2214, -132.602) knots 0 0 0 1 1 1
  line L929 (69.2214, -132.602) -> (69.2214, -119.3804)
  spline S1101 degree 2 poles (69.2214, -119.3804) (69.2214, -118.3269) (68.4664, -117.5719) knots 0 0 0 1 1 1
  spline S1102 degree 2 poles (68.4664, -117.5719) (68.3259, -117.4314) (68.1679, -117.3085) knots 0 0 0 1 1 1
  spline S1103 degree 2 poles (64.3577, -110.3729) (64.8845, -110.3729) (65.6395, -111.1279) (65.6395, -111.6547) knots 0 0 0 1 2 2 2
  spline S1104 degree 2 poles (65.6395, -111.6547) (65.6395, -112.1814) (64.8845, -112.9189) (64.3577, -112.9189) knots 0 0 0 1 2 2 2
  spline S1105 degree 2 poles (64.3577, -112.9189) (63.831, -112.9189) (63.0935, -112.1814) (63.0935, -111.6547) knots 0 0 0 1 2 2 2
  spline S1106 degree 2 poles (63.0935, -111.6547) (63.0935, -111.1279) (63.831, -110.3729) (64.3577, -110.3729) knots 0 0 0 1 2 2 2
  spline S1107 degree 2 poles (68.9932, -110.3729) (69.5199, -110.3729) (70.2574, -111.1279) (70.2574, -111.6547) knots 0 0 0 1 2 2 2
  spline S1108 degree 2 poles (70.2574, -111.6547) (70.2574, -112.1814) (69.5199, -112.9189) (68.9932, -112.9189) knots 0 0 0 1 2 2 2
  spline S1109 degree 2 poles (68.9932, -112.9189) (68.4664, -112.9189) (67.7114, -112.1814) (67.7114, -111.6547) knots 0 0 0 1 2 2 2
  spline S1110 degree 2 poles (67.7114, -111.6547) (67.7114, -111.1279) (68.4664, -110.3729) (68.9932, -110.3729) knots 0 0 0 1 2 2 2
  spline S1111 degree 2 poles (95.5489, -116.1497) (95.5489, -115.7458) (96.1108, -115.1839) (96.4971, -115.1839) knots 0 0 0 1 2 2 2
  spline S1112 degree 2 poles (96.4971, -115.1839) (96.9009, -115.1839) (97.4628, -115.7458) (97.4628, -116.1497) knots 0 0 0 1 2 2 2
  line L930 (97.4628, -116.1497) -> (97.4628, -132.0401)
  spline S1113 degree 2 poles (97.4628, -132.0401) (97.4628, -133.0936) (98.9553, -134.5861) (100.0088, -134.5861) knots 0 0 0 1 2 2 2
  spline S1114 degree 2 poles (100.0088, -134.5861) (101.0623, -134.5861) (102.5548, -133.0936) (102.5548, -132.0401) knots 0 0 0 1 2 2 2
  line L931 (102.5548, -132.0401) -> (102.5548, -116.1497)
  spline S1115 degree 2 poles (102.5548, -116.1497) (102.5548, -115.7458) (103.0991, -115.1839) (103.5029, -115.1839) knots 0 0 0 1 2 2 2
  spline S1116 degree 2 poles (103.5029, -115.1839) (103.9068, -115.1839) (104.4686, -115.7458) (104.4686, -116.1497) knots 0 0 0 1 2 2 2
  line L932 (104.4686, -116.1497) -> (104.4686, -132.0401)
  spline S1117 degree 2 poles (104.4686, -132.0401) (104.4686, -133.8838) (101.8524, -136.5) (100.0088, -136.5) knots 0 0 0 1 2 2 2
  spline S1118 degree 2 poles (100.0088, -136.5) (98.1651, -136.5) (95.5489, -133.8838) (95.5489, -132.0401) knots 0 0 0 1 2 2 2
  line L933 (95.5489, -132.0401) -> (95.5489, -116.1497)
  spline S1119 degree 2 poles (136.5114, -125.0343) (136.9153, -125.0343) (137.4771, -125.5962) (137.4771, -126) knots 0 0 0 1 2 2 2
  spline S1120 degree 2 poles (137.4771, -126) (137.4771, -126.3863) (136.9153, -126.9482) (136.5114, -126.9482) knots 0 0 0 1 2 2 2
  line L934 (136.5114, -126.9482) -> (132.3852, -126.9482)
  line L935 (132.3852, -126.9482) -> (132.3852, -135.5518)
  spline S1121 degree 2 poles (132.3852, -135.5518) (132.3852, -135.9381) (131.8233, -136.5) (131.4195, -136.5) knots 0 0 0 1 2 2 2
  spline S1122 degree 2 poles (131.4195, -136.5) (131.0332, -136.5) (130.4713, -135.9381) (130.4713, -135.5518) knots 0 0 0 1 2 2 2
  line L936 (130.4713, -135.5518) -> (130.4713, -116.4482)
  spline S1123 degree 2 poles (130.4713, -116.4482) (130.4713, -116.0443) (131.0332, -115.5) (131.4195, -115.5) knots 0 0 0 1 2 2 2
  line L937 (131.4195, -115.5) -> (137.4947, -115.5)
  spline S1124 degree 2 poles (137.4947, -115.5) (137.881, -115.5) (138.4429, -116.0443) (138.4429, -116.4482) knots 0 0 0 1 2 2 2
  spline S1125 degree 2 poles (138.4429, -116.4482) (138.4429, -116.8344) (137.881, -117.3963) (137.4947, -117.3963) knots 0 0 0 1 2 2 2
  line L938 (137.4947, -117.3963) -> (132.3852, -117.3963)
  line L939 (132.3852, -117.3963) -> (132.3852, -125.0343)
  line L940 (132.3852, -125.0343) -> (136.5114, -125.0343)
  spline S1126 degree 2 poles (165.7097, -116.4482) (165.7097, -116.0443) (166.2716, -115.5) (166.6579, -115.5) knots 0 0 0 1 2 2 2
  spline S1127 degree 2 poles (166.6579, -115.5) (167.0617, -115.5) (167.6236, -116.0443) (167.6236, -116.4482) knots 0 0 0 1 2 2 2
  line L941 (167.6236, -116.4482) -> (167.6236, -135.5518)
  spline S1128 degree 2 poles (167.6236, -135.5518) (167.6236, -135.9381) (167.0617, -136.5) (166.6579, -136.5) knots 0 0 0 1 2 2 2
  spline S1129 degree 2 poles (166.6579, -136.5) (166.2716, -136.5) (165.7097, -135.9381) (165.7097, -135.5518) knots 0 0 0 1 2 2 2
  line L942 (165.7097, -135.5518) -> (165.7097, -116.4482)
  spline S1130 degree 2 poles (-170.4417, -153.3963) (-170.8456, -153.3963) (-171.4075, -152.852) (-171.4075, -152.4482) knots 0 0 0 1 2 2 2
  spline S1131 degree 2 poles (-171.4075, -152.4482) (-171.4075, -152.0443) (-170.8456, -151.5) (-170.4417, -151.5) knots 0 0 0 1 2 2 2
  line L943 (-170.4417, -151.5) -> (-163.1198, -151.5)
  spline S1132 degree 2 poles (-163.1198, -151.5) (-162.7336, -151.5) (-162.1717, -152.0443) (-162.1717, -152.4482) knots 0 0 0 1 2 2 2
  spline S1133 degree 2 poles (-162.1717, -152.4482) (-162.1717, -152.6413) (-162.2419, -152.8169) knots 0 0 0 1 1 1
  line L944 (-162.2419, -152.8169) -> (-169.0546, -170.5861)
  line L945 (-169.0546, -170.5861) -> (-163.1198, -170.5861)
  spline S1134 degree 2 poles (-163.1198, -170.5861) (-162.7336, -170.5861) (-162.1717, -171.148) (-162.1717, -171.5518) knots 0 0 0 1 2 2 2
  spline S1135 degree 2 poles (-162.1717, -171.5518) (-162.1717, -171.9206) (-162.7336, -172.5) (-163.1198, -172.5) knots 0 0 0 1 2 2 2
  line L946 (-163.1198, -172.5) -> (-170.4417, -172.5)
  spline S1136 degree 2 poles (-170.4417, -172.5) (-170.828, -172.5) (-171.3899, -171.9206) (-171.3899, -171.5518) knots 0 0 0 1 2 2 2
  spline S1137 degree 2 poles (-171.3899, -171.5518) (-171.3899, -171.306) (-171.3021, -171.1129) knots 0 0 0 1 1 1
  line L947 (-171.3021, -171.1129) -> (-164.5245, -153.3963)
  line L948 (-164.5245, -153.3963) -> (-170.4417, -153.3963)
  spline S1138 degree 2 poles (-128.496, -171.6747) (-128.5486, -171.9732) (-128.7769, -172.2191) knots 0 0 0 1 1 1
  spline S1139 degree 2 poles (-128.7769, -172.2191) (-129.0578, -172.5) (-129.4441, -172.5) knots 0 0 0 1 1 1
  spline S1140 degree 2 poles (-129.4441, -172.5) (-129.848, -172.5) (-130.1113, -172.2191) knots 0 0 0 1 1 1
  spline S1141 degree 2 poles (-130.1113, -172.2191) (-130.322, -171.9732) (-130.3747, -171.6747) knots 0 0 0 1 1 1
  line L949 (-130.3747, -171.6747) -> (-133.3421, -159.6472)
  line L950 (-133.3421, -159.6472) -> (-136.2919, -171.6572)
  spline S1142 degree 2 poles (-136.2919, -171.6572) (-136.3446, -171.9732) (-136.5729, -172.2191) knots 0 0 0 1 1 1
  spline S1143 degree 2 poles (-136.5729, -172.2191) (-136.8538, -172.5) (-137.2401, -172.5) knots 0 0 0 1 1 1
  spline S1144 degree 2 poles (-137.2401, -172.5) (-137.644, -172.5) (-137.9073, -172.2191) knots 0 0 0 1 1 1
  spline S1145 degree 2 poles (-137.9073, -172.2191) (-138.1356, -171.9732) (-138.2058, -171.6747) knots 0 0 0 1 1 1
  line L951 (-138.2058, -171.6747) -> (-142.7886, -152.6589)
  spline S1146 degree 2 poles (-142.7886, -152.6589) (-142.8062, -152.5535) (-142.8062, -152.4482) knots 0 0 0 1 1 1
  spline S1147 degree 2 poles (-142.8062, -152.4482) (-142.8062, -152.0443) (-142.2618, -151.5) (-141.858, -151.5) knots 0 0 0 1 2 2 2
  spline S1148 degree 2 poles (-141.858, -151.5) (-141.4542, -151.5) (-141.1732, -151.7634) knots 0 0 0 1 1 1
  spline S1149 degree 2 poles (-141.1732, -151.7634) (-140.9625, -151.9916) (-140.9098, -152.2901) knots 0 0 0 1 1 1
  line L952 (-140.9098, -152.2901) -> (-137.2401, -167.4607)
  line L953 (-137.2401, -167.4607) -> (-134.3605, -155.6263)
  spline S1150 degree 2 poles (-134.3605, -155.6263) (-134.2552, -155.1873) (-133.7284, -154.6781) (-133.3246, -154.6781) knots 0 0 0 1 2 2 2
  spline S1151 degree 2 poles (-133.3246, -154.6781) (-132.9207, -154.6781) (-132.4115, -155.2224) (-132.3237, -155.6263) knots 0 0 0 1 2 2 2
  line L954 (-132.3237, -155.6263) -> (-129.4441, -167.4607)
  line L955 (-129.4441, -167.4607) -> (-125.7744, -152.2901)
  spline S1152 degree 2 poles (-125.7744, -152.2901) (-125.7217, -151.9916) (-125.4935, -151.7634) knots 0 0 0 1 1 1
  spline S1153 degree 2 poles (-125.4935, -151.7634) (-125.2301, -151.5) (-124.8262, -151.5) knots 0 0 0 1 1 1
  spline S1154 degree 2 poles (-124.8262, -151.5) (-124.4224, -151.5) (-123.8781, -152.0443) (-123.8781, -152.4482) knots 0 0 0 1 2 2 2
  spline S1155 degree 2 poles (-123.8781, -152.4482) (-123.8781, -152.5535) (-123.8956, -152.6589) knots 0 0 0 1 1 1
  line L956 (-123.8956, -152.6589) -> (-128.496, -171.6747)
  spline S1156 degree 2 poles (-102.467, -151.6405) (-102.2212, -151.4824) (-101.9051, -151.4824) knots 0 0 0 1 1 1
  spline S1157 degree 2 poles (-101.9051, -151.4824) (-101.5188, -151.4824) (-100.9569, -152.0443) (-100.9569, -152.4306) knots 0 0 0 1 2 2 2
  spline S1158 degree 2 poles (-100.9569, -152.4306) (-100.9569, -152.8344) (-101.2203, -153.0978) knots 0 0 0 1 1 1
  spline S1159 degree 2 poles (-101.2203, -153.0978) (-101.3081, -153.1681) (-101.3783, -153.2383) knots 0 0 0 1 1 1
  spline S1160 degree 2 poles (-101.3783, -153.2383) (-101.6066, -153.3788) (-101.7997, -153.5719) knots 0 0 0 1 1 1
  spline S1161 degree 2 poles (-101.7997, -153.5719) (-102.5372, -154.3269) (-102.5372, -155.3804) knots 0 0 0 1 1 1
  line L957 (-102.5372, -155.3804) -> (-102.5372, -168.602)
  spline S1162 degree 2 poles (-102.5372, -168.602) (-102.5372, -169.6555) (-101.7997, -170.393) knots 0 0 0 1 1 1
  spline S1163 degree 2 poles (-101.7997, -170.393) (-101.6066, -170.5861) (-101.3783, -170.7266) knots 0 0 0 1 1 1
  spline S1164 degree 2 poles (-101.3783, -170.7266) (-101.3081, -170.7793) (-101.2379, -170.8495) knots 0 0 0 1 1 1
  spline S1165 degree 2 poles (-101.2379, -170.8495) (-100.9569, -171.1304) (-100.9569, -171.5343) knots 0 0 0 1 1 1
  spline S1166 degree 2 poles (-100.9569, -171.5343) (-100.9569, -171.9206) (-101.5188, -172.4824) (-101.9051, -172.4824) knots 0 0 0 1 2 2 2
  spline S1167 degree 2 poles (-101.9051, -172.4824) (-102.2036, -172.4824) (-102.4319, -172.342) knots 0 0 0 1 1 1
  spline S1168 degree 2 poles (-102.4319, -172.342) (-102.8181, -172.0786) (-103.1518, -171.745) knots 0 0 0 1 1 1
  spline S1169 degree 2 poles (-103.1518, -171.745) (-104.4511, -170.4457) (-104.4511, -168.602) knots 0 0 0 1 1 1
  line L958 (-104.4511, -168.602) -> (-104.4511, -155.3804)
  spline S1170 degree 2 poles (-104.4511, -155.3804) (-104.4511, -153.5192) (-103.1518, -152.2199) knots 0 0 0 1 1 1
  spline S1171 degree 2 poles (-103.1518, -152.2199) (-102.8181, -151.8863) (-102.467, -151.6405) knots 0 0 0 1 1 1
  spline S1172 degree 2 poles (-98.4987, -153.3085) (-98.6392, -153.2383) (-98.7621, -153.1154) knots 0 0 0 1 1 1
  spline S1173 degree 2 poles (-98.7621, -153.1154) (-99.0431, -152.8344) (-99.0431, -152.4482) knots 0 0 0 1 1 1
  spline S1174 degree 2 poles (-99.0431, -152.4482) (-99.0431, -152.0443) (-98.4812, -151.4824) (-98.0949, -151.4824) knots 0 0 0 1 2 2 2
  spline S1175 degree 2 poles (-98.0949, -151.4824) (-97.7788, -151.4824) (-97.5155, -151.658) knots 0 0 0 1 1 1
  spline S1176 degree 2 poles (-97.5155, -151.658) (-97.1643, -151.9038) (-96.8482, -152.2199) knots 0 0 0 1 1 1
  spline S1177 degree 2 poles (-96.8482, -152.2199) (-95.5489, -153.5192) (-95.5489, -155.3804) knots 0 0 0 1 1 1
  line L959 (-95.5489, -155.3804) -> (-95.5489, -168.602)
  spline S1178 degree 2 poles (-95.5489, -168.602) (-95.5489, -170.4457) (-96.8482, -171.745) knots 0 0 0 1 1 1
  spline S1179 degree 2 poles (-96.8482, -171.745) (-97.1994, -172.0962) (-97.5857, -172.3595) knots 0 0 0 1 1 1
  spline S1180 degree 2 poles (-97.5857, -172.3595) (-97.7964, -172.5) (-98.0949, -172.5) knots 0 0 0 1 1 1
  spline S1181 degree 2 poles (-98.0949, -172.5) (-98.4812, -172.5) (-99.0431, -171.9206) (-99.0431, -171.5518) knots 0 0 0 1 2 2 2
  spline S1182 degree 2 poles (-99.0431, -171.5518) (-99.0431, -171.148) (-98.7621, -170.8671) knots 0 0 0 1 1 1
  spline S1183 degree 2 poles (-98.7621, -170.8671) (-98.6919, -170.7968) (-98.6217, -170.7441) knots 0 0 0 1 1 1
  spline S1184 degree 2 poles (-98.6217, -170.7441) (-98.411, -170.6037) (-98.2003, -170.393) knots 0 0 0 1 1 1
  spline S1185 degree 2 poles (-98.2003, -170.393) (-97.4452, -169.6555) (-97.4452, -168.602) knots 0 0 0 1 1 1
  line L960 (-97.4452, -168.602) -> (-97.4452, -155.3804)
  spline S1186 degree 2 poles (-97.4452, -155.3804) (-97.4452, -154.3269) (-98.2003, -153.5719) knots 0 0 0 1 1 1
  spline S1187 degree 2 poles (-98.2003, -153.5719) (-98.3407, -153.4314) (-98.4987, -153.3085) knots 0 0 0 1 1 1
  spline S1188 degree 2 poles (-97.6735, -146.3729) (-97.1467, -146.3729) (-96.4093, -147.1279) (-96.4093, -147.6547) knots 0 0 0 1 2 2 2
  spline S1189 degree 2 poles (-96.4093, -147.6547) (-96.4093, -148.1814) (-97.1467, -148.9189) (-97.6735, -148.9189) knots 0 0 0 1 2 2 2
  spline S1190 degree 2 poles (-97.6735, -148.9189) (-98.2003, -148.9189) (-98.9553, -148.1814) (-98.9553, -147.6547) knots 0 0 0 1 2 2 2
  spline S1191 degree 2 poles (-98.9553, -147.6547) (-98.9553, -147.1279) (-98.2003, -146.3729) (-97.6735, -146.3729) knots 0 0 0 1 2 2 2
  spline S1192 degree 2 poles (-102.3089, -146.3729) (-101.7822, -146.3729) (-101.0272, -147.1279) (-101.0272, -147.6547) knots 0 0 0 1 2 2 2
  spline S1193 degree 2 poles (-101.0272, -147.6547) (-101.0272, -148.1814) (-101.7822, -148.9189) (-102.3089, -148.9189) knots 0 0 0 1 2 2 2
  spline S1194 degree 2 poles (-102.3089, -148.9189) (-102.8357, -148.9189) (-103.5732, -148.1814) (-103.5732, -147.6547) knots 0 0 0 1 2 2 2
  spline S1195 degree 2 poles (-103.5732, -147.6547) (-103.5732, -147.1279) (-102.8357, -146.3729) (-102.3089, -146.3729) knots 0 0 0 1 2 2 2
  spline S1196 degree 2 poles (-71.1178, -152.1497) (-71.1178, -151.7458) (-70.5559, -151.1839) (-70.1696, -151.1839) knots 0 0 0 1 2 2 2
  spline S1197 degree 2 poles (-70.1696, -151.1839) (-69.7657, -151.1839) (-69.2039, -151.7458) (-69.2039, -152.1497) knots 0 0 0 1 2 2 2
  line L961 (-69.2039, -152.1497) -> (-69.2039, -168.0401)